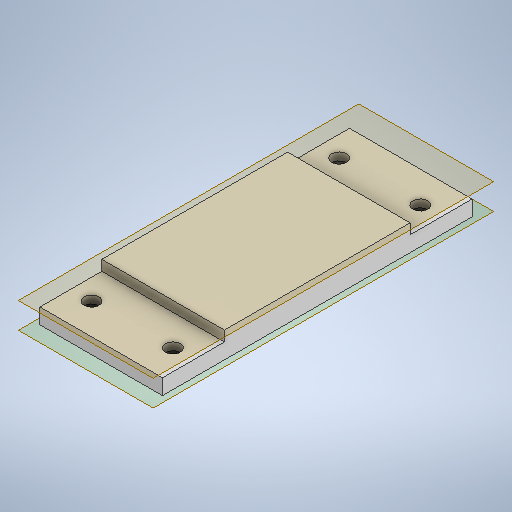
# Autodesk Inventor part: motor_rot_born2
Saved by Autodesk Inventor 2025.2 (Build 292293000, 293)
## iProperties
Created: 2024-12-22
Part Number: motor_rot_born2
Material: 一般
Document SubType Name: Modeling
Designer: mahhy
Density: 1 g/cm^3
Appearance: 既定
Author: mahhy
Autodesk Inventor part; units mm, degrees
ref_plane "YZ Plane" through (0, 0, 0) normal (1, 0, 0) x (0, 1, 0)
ref_plane "XZ Plane" through (0, 0, 0) normal (0, 1, 0) x (-1, 0, 0)
ref_plane "XY Plane" through (0, 0, 0) normal (0, 0, 1) x (1, 0, 0)
sketch "スケッチ1" plane through (0, 0, 0) normal (0, 1, 0) x (-1, 0, 0)
  line L0 (0, 0) -> (47.5, 0)
  line L1 (47.5, 0) -> (47.5, -120)
  line L2 (47.5, -120) -> (0, -120)
  line L3 (0, -120) -> (0, 0)
  dimension "d0" = 47.5
  dimension "d1" = 120
  constraints: 8 end point, 2 parallel, 1 horizontal, 1 perpendicular
  measures "d0" distance of L1.end L2.end
  measures "d1" distance of L0.end L1.end
extrude "押し出し1" add sketch "スケッチ1" along normal blind 10
ref_plane "作業平面1" through (0, 10, 0) normal (0, 1, 0) x (1, 0, 0)
sketch "スケッチ2" plane through (0, 10, 0) normal (0, 1, 0) x (1, 0, 0)
  line L0 (0, 120) -> (-47.5, 120) projected
  line L1 (0, 0) -> (0, 120) projected
  line L2 (-47.5, 120) -> (0, 120)
  line L3 (0, 120) -> (0, 96)
  line L4 (0, 96) -> (-47.5, 96)
  line L5 (-47.5, 96) -> (-47.5, 120)
  line L6 (-47.5, 120) -> (-47.5, 0) projected
  line L7 (0, 0) -> (-47.5, 0)
  line L8 (-47.5, 0) -> (-47.5, 24)
  line L9 (-47.5, 24) -> (0, 24)
  line L10 (0, 24) -> (0, 0)
  point P0 (0, 24)
  dimension "d5" = 24
  dimension "d6" = 24
  dimension "d7" = 72
  constraints: 16 end point, 4 parallel, 2 horizontal, 2 perpendicular, 2 point on line
  measures "d5" distance of L2.end L3.end
  measures "d6" distance of L7.end L8.end
  measures "d7" distance between parallel lines of L4 L9
extrude "押し出し2" cut sketch "スケッチ2" against normal blind 4 contours L1 L4 L5 L0 | L1 L7 L6 L9
ref_plane "作業平面2" through (0, 0, 0) normal (0, -1, 0) x (1, 0, 0)
sketch "スケッチ3" plane through (0, 0, 0) normal (0, -1, 0) x (1, 0, 0)
  line L0 (-47.5, 0) -> (0, 0) projected
  line L1 (0, -120) -> (-47.5, -120) projected
  line L2 (-47.5, -120) -> (-47.5, 0) projected
  line L3 (0, 0) -> (0, -120) projected
  point P0 (-39.5, -12)
  point P1 (-8, -12)
  point P2 (-39.5, -108)
  point P3 (-8, -108)
  dimension "d11" = 12
  dimension "d12" = 12
  dimension "d13" = 12
  dimension "d14" = 12
  dimension "d15" = 8
  dimension "d16" = 8
  dimension "d17" = 8
  dimension "d18" = 8
  measures "d11" distance from line of L0 point (-39.5, -12)
  measures "d12" distance from line of L0 point (-8, -12)
  measures "d13" distance from line of L1 point (-8, -108)
  measures "d14" distance from line of L1 point (-39.5, -108)
  measures "d15" distance from line of L2 point (-39.5, -12)
  measures "d16" distance from line of L3 point (-8, -12)
  measures "d17" distance from line of L2 point (-39.5, -108)
  measures "d18" distance from line of L3 point (-8, -108)
hole "穴1" at (-39.5, 0, -12) at (-8, 0, -12) at (-39.5, 0, -108) at (-8, 0, -108) direction (0, 1, 0) diameter 5.8 depth 7
sketch "スケッチ4" plane through (0, 0, 0) normal (0, -1, 0) x (1, 0, 0)
  circle A0 centre (-8, -12) radius 2.9 projected
  circle A1 centre (-8, -12) radius 4.5
  circle A2 centre (-39.5, -12) radius 2.9 projected
  circle A3 centre (-39.5, -12) radius 4.5
  circle A4 centre (-39.5, -108) radius 2.9 projected
  circle A5 centre (-39.5, -108) radius 4.5
  circle A6 centre (-8, -108) radius 2.9 projected
  circle A7 centre (-8, -108) radius 4.5
  point P0 (0, 0)
  dimension "d26" = 9
  dimension "d27" = 9
  dimension "d28" = 9
  dimension "d29" = 9
  constraints: 4 centre point, 4 coincident
  measures "d26" diameter of A1
  measures "d27" diameter of A3
  measures "d28" diameter of A5
  measures "d29" diameter of A7
extrude "押し出し3" cut sketch "スケッチ4" against normal blind 3
